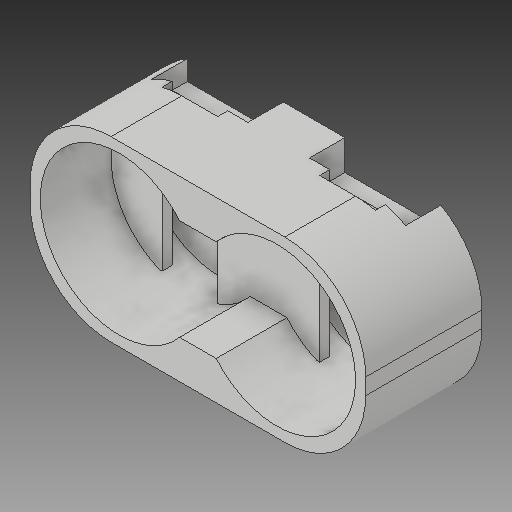
# Autodesk Inventor part: CaseBottom_CR123A
Saved by Autodesk Inventor 2018.1 (Build 221171000, 171)
## iProperties
Created: 2017-09-02
Part Number: CaseBottom_CR123A
Material: 一般
Document SubType Name: Modeling
Designer: sktom
Density: 1 g/cm^3
Appearance: 既定
Author: sktom
Autodesk Inventor part; units mm, degrees
ref_plane "YZ Plane" through (0, 0, 0) normal (1, 0, 0) x (0, 1, 0)
ref_plane "XZ Plane" through (0, 0, 0) normal (0, 1, 0) x (-1, 0, 0)
ref_plane "XY Plane" through (0, 0, 0) normal (0, 0, 1) x (1, 0, 0)
sketch "スケッチ4" plane through (0, 0, 0) normal (0, 0, 1) x (1, 0, 0)
  circle A0 centre (-7.8, 0) radius 7.8
  circle A1 centre (7.8, 0) radius 7.8
  line L0 (-15.6, -7.8) -> (15.6, -7.8)
  line L1 (15.6, -7.8) -> (15.6, 7.8)
  line L2 (15.6, 7.8) -> (-15.6, 7.8)
  line L3 (-15.6, 7.8) -> (-15.6, -7.8)
  line L4 (-16.6, 8.8) -> (16.6, 8.8)
  line L5 (16.6, 8.8) -> (16.6, -8.8)
  line L6 (16.6, -8.8) -> (-16.6, -8.8)
  line L7 (-16.6, -8.8) -> (-16.6, 8.8)
  line L8 (-1.8133, 5) -> (1.8133, 5)
  line L9 (-1.8133, -5) -> (1.8133, -5)
  point P0 (0, 0)
  dimension "d12" = 15.6
  dimension "d13" = 1
  dimension "d14" = 10
  constraints: 20 end point, 7 parallel, 5 point on circle, 5 tangent, 2 centre point, 2 horizontal alignment, 2 perpendicular, 1 equal radius, 1 horizontal, 3 other
  measures "d12" diameter of A1
  measures "d13" distance between parallel lines of L2 L4
  measures "d14" distance between parallel lines of L8 L9
extrude "押し出し4" add sketch "スケッチ4" along normal blind 10 contours A0 L2 A1 L8 | L9 A1 L0 A0 | A0 L3 L2 | L0 L3 A0 | L2 L1 A1 | A1 L1 L0 | L4 L5 L6 L7
sketch "スケッチ5" plane through (0, 0, 0) normal (0, 0, -1) x (-1, 0, 0)
  arc A0 (-1.8133, 5) -> (-1.8133, -5) centre (-7.8, 0) ccw projected
  line L0 (-1.8133, 5) -> (1.8133, 5) projected
  arc A1 (1.8133, -5) -> (1.8133, 5) centre (7.8, 0) ccw projected
  line L1 (1.8133, -5) -> (-1.8133, -5) projected
  line L2 (16.6, 8.8) -> (-16.6, 8.8) projected
  line L3 (-16.6, 8.8) -> (-16.6, -8.8) projected
  line L4 (-16.6, -8.8) -> (16.6, -8.8) projected
  line L5 (16.6, -8.8) -> (16.6, 8.8) projected
  point P0 (0, 0)
extrude "押し出し5" add sketch "スケッチ5" along normal blind 1.5 contours L0 A1 L1 A0 | L5 L4 L3 L2
sketch "スケッチ6" plane through (-16.6, 8.8, 10) normal (0, 1, 0) x (1, 0, 0)
  line L0 (14.7867, 10) -> (14.7867, 10) construction
  line L1 (14.7867, 10) -> (14.7867, 0) construction
  line L2 (14.7867, 0) -> (14.7867, 0) construction
  line L3 (14.7867, 10) -> (14.7867, 0) construction
  line L4 (18.4133, 10) -> (18.4133, 10) construction
  line L5 (18.4133, 10) -> (18.4133, 0) construction
  line L6 (18.4133, 0) -> (18.4133, 0) construction
  line L7 (18.4133, 10) -> (18.4133, 0) construction
  line L8 (18.4133, 10) -> (18.4133, 10) construction
  line L9 (18.4133, 10) -> (14.7867, 10) construction
  line L10 (14.7867, 10) -> (14.7867, 10) construction
  line L11 (14.7867, 10) -> (18.4133, 10) construction
  line L12 (14.7867, 10) -> (1, 10) construction
  line L13 (1, 10) -> (1, 8) construction
  line L14 (1, 8) -> (16.6, 8) construction
  line L15 (14.7867, 8) -> (14.7867, 10) construction
  line L16 (32.2, 10) -> (32.2, 0) construction
  line L17 (18.4133, 10) -> (32.2, 10) construction
  line L18 (32.2, 10) -> (32.2, 8) construction
  line L19 (32.2, 8) -> (16.6, 8) construction
  line L20 (18.4133, 7.5) -> (18.4133, 10) construction
  line L21 (4.05, 10) -> (13.55, 10)
  line L22 (13.55, 10) -> (13.55, 8)
  line L23 (13.55, 8) -> (4.05, 8)
  line L24 (4.05, 8) -> (4.05, 10)
  line L25 (18.4133, 10) -> (32.2, 10) projected
  line L26 (19.65, 10) -> (29.15, 10)
  line L27 (29.15, 10) -> (29.15, 8)
  line L28 (29.15, 8) -> (19.65, 8)
  line L29 (19.65, 8) -> (19.65, 10)
  line L30 (1, 10) -> (16.6, 10)
  line L31 (16.6, 10) -> (16.6, 7)
  line L32 (16.6, 7) -> (1, 7)
  line L33 (1, 7) -> (1, 10)
  line L34 (32.2, 10) -> (16.6, 10)
  line L35 (16.6, 10) -> (16.6, 7)
  line L36 (16.6, 7) -> (32.2, 7)
  line L37 (32.2, 7) -> (32.2, 10)
  line L38 (6.05, 8) -> (11.55, 8)
  line L39 (11.55, 8) -> (11.55, 7)
  line L40 (11.55, 7) -> (6.05, 7)
  line L41 (6.05, 7) -> (6.05, 8)
  line L42 (21.65, 8) -> (27.15, 8)
  line L43 (27.15, 8) -> (27.15, 7)
  line L44 (27.15, 7) -> (21.65, 7)
  line L45 (21.65, 7) -> (21.65, 8)
  point P0 (16.6, 10)
  point P1 (24.4, 8)
  point P2 (8.8, 8)
  dimension "d19" = 2
  dimension "d20" = 9.5
  dimension "d21" = 1
  dimension "d22" = 5.5
  constraints: 64 end point, 16 parallel, 14 point on line, 8 horizontal, 8 midpoint, 8 perpendicular, 4 collinear
  measures "d19" distance between parallel lines of L14 L12
  measures "d20" distance of L22.end L23.end
  measures "d21" distance between parallel lines of L19 L36
  measures "d22" distance of L38.start L38.end
extrude "押し出し6" cut sketch "スケッチ6" against normal blind 15 contours L21 L22 L23 L24 | L23 L39 L32 L41 | L45 L28 L43 L36 | L25 L27 L28 L29
extrude "押し出し7" add sketch "スケッチ6" against normal blind 16 contours L24 L23 L41 L32 L33 L30 | L30 L31 L32 L39 L23 L22 | L34 L25 L29 L28 L45 L36 L31 | L43 L28 L27 L25 L37 L36
sketch "スケッチ7" plane through (0, 0, -1.5) normal (0, 0, -1) x (-1, 0, 0)
  line L0 (12.55, 8.8) -> (12.55, -6.2) construction
  line L1 (3.05, 8.8) -> (3.05, -6.2) construction
  line L2 (12.55, 8.8) -> (3.05, 8.8) construction
  line L3 (-12.55, 8.8) -> (-12.55, -6.2) construction
  line L4 (-3.05, 8.8) -> (-12.55, 8.8) construction
  line L5 (-3.05, 8.8) -> (-3.05, -6.2) construction
  line L6 (-3.05, 8.8) -> (-3.05, -6.2) projected
  line L7 (-12.55, 8.8) -> (-3.05, 8.8)
  line L8 (-3.05, 8.8) -> (-3.05, 5.8)
  line L9 (-3.05, 5.8) -> (-12.55, 5.8)
  line L10 (-12.55, 5.8) -> (-12.55, 8.8)
  line L11 (3.05, 8.8) -> (12.55, 8.8)
  line L12 (12.55, 8.8) -> (12.55, 5.8)
  line L13 (12.55, 5.8) -> (3.05, 5.8)
  line L14 (3.05, 5.8) -> (3.05, 8.8)
  line L15 (-3.05, -6.2) -> (-3.0671, -6.2) projected
  arc A0 (-12.5329, -6.2) -> (-3.0671, -6.2) centre (-7.8, 0) ccw projected
  line L16 (-12.5329, -6.2) -> (-12.55, -6.2) projected
  line L17 (12.55, -6.2) -> (12.5329, -6.2) projected
  arc A1 (3.0671, -6.2) -> (12.5329, -6.2) centre (7.8, 0) ccw projected
  line L18 (3.0671, -6.2) -> (3.05, -6.2) projected
  point P0 (0, 0)
  point P1 (-3.05, -5.2)
  dimension "d27" = 3
  constraints: 16 end point, 4 parallel, 3 point on line, 2 horizontal, 2 perpendicular
  measures "d27" distance between parallel lines of L2 L13
extrude "押し出し8" cut sketch "スケッチ7" against normal up to next
fillet "フィレット1" radius 8 4 edges at (16.6, 8.8, 4.25) (16.6, -8.8, 4.25) (-16.6, 8.8, 4.25) (-16.6, -8.8, 4.25)
